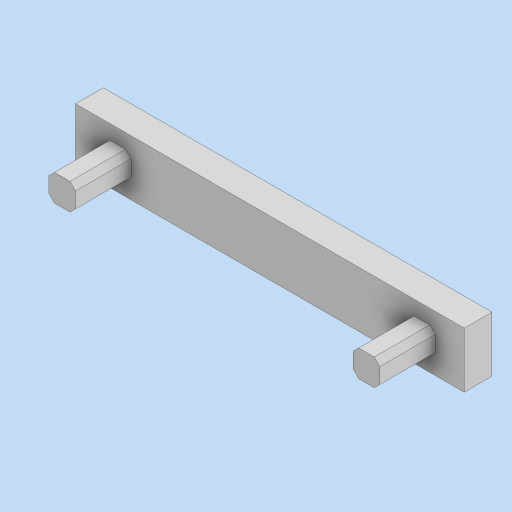
# Autodesk Inventor part: UNION_INTERNA
Saved by Autodesk Inventor 2024 (Build 280153000, 153)
## iProperties
Created: 2024-11-05
Part Number: UNION_INTERNA
Material: Generic
Document SubType Name: Modeling
Designer: MxMon
Density: 1 g/cm^3
Appearance: Default
Author: MxMon
Autodesk Inventor part; units mm, degrees
ref_plane "YZ Plane" through (0, 0, 0) normal (1, 0, 0) x (0, 1, 0)
ref_plane "XZ Plane" through (0, 0, 0) normal (0, 1, 0) x (-1, 0, 0)
ref_plane "XY Plane" through (0, 0, 0) normal (0, 0, 1) x (1, 0, 0)
sketch "Sketch1" plane through (0, 0, 0) normal (0, 0, 1) x (1, 0, 0)
  line L0 (-35, 5) -> (35, 5)
  line L1 (35, 5) -> (35, -5)
  line L2 (35, -5) -> (-35, -5)
  line L3 (-35, -5) -> (-35, 5)
  line L4 (-35, 5) -> (35, -5) construction
  line L5 (35, 5) -> (-35, -5) construction
  point P0 (0, 0)
  dimension "d0" = 70
  dimension "d1" = 10
  constraints: 12 end point, 2 midpoint, 2 parallel, 1 horizontal, 1 perpendicular
  measures "d0" distance of L1.end L2.end
  measures "d1" distance of L0.end L1.end
extrude "Extrusion1" add sketch "Sketch1" along normal blind 5
sketch "Sketch2" plane through (0, 0, 5) normal (0, 0, 1) x (1, 0, 0)
  line L0 (-29.8, 2.4) -> (-25, 2.4)
  line L1 (-25, 2.4) -> (-25, -2.4)
  line L2 (-25, -2.4) -> (-29.8, -2.4)
  line L3 (-29.8, -2.4) -> (-29.8, 2.4)
  line L4 (-29.8, 2.4) -> (-25, -2.4) construction
  line L5 (-25, 2.4) -> (-29.8, -2.4) construction
  line L6 (35, 5) -> (-35, 5) construction
  line L7 (-35, -5) -> (35, -5) construction
  line L8 (0, 5) -> (0, -5) construction
  line L9 (29.8, 2.4) -> (25, 2.4)
  line L10 (25, 2.4) -> (25, -2.4)
  line L11 (25, -2.4) -> (29.8, -2.4)
  line L12 (29.8, -2.4) -> (29.8, 2.4)
  point P0 (0, 0)
  point P1 (-27.4, 0)
  point P2 (-25, 0)
  dimension "d4" = 4.8
  dimension "d5" = 4.8
  dimension "d6" = 25
  constraints: 22 end point, 5 midpoint, 4 symmetric about line, 2 parallel, 1 horizontal, 1 horizontal alignment, 1 perpendicular
  measures "d4" distance of L1.end L2.end
  measures "d5" distance of L0.end L1.end
  measures "d6" horizontal distance of L0.end point (0, 0)
extrude "Extrusion2" add sketch "Sketch2" along normal blind 10
chamfer "Chamfer1" distance 1 angle 45 8 edges at (-29.8, 2.4, 10) (-25, 2.4, 10) (-29.8, -2.4, 10) (-25, -2.4, 10) (25, 2.4, 10) (29.8, 2.4, 10) (29.8, -2.4, 10) (25, -2.4, 10)
body "Solid1"
